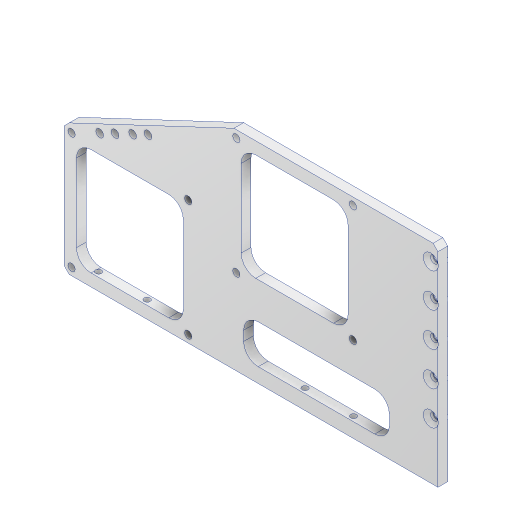
# Autodesk Inventor part: 사이드프레임
Saved by Autodesk Inventor 2023.2 (Build 272271000, 271)
## iProperties
Created: 2022-12-27
Part Number: 사이드프레임
Material: 알루미늄 6061
Document SubType Name: Modeling
Designer: BAEK
Density: 2.7 g/cm^3
Appearance: 알루미늄 - 평지
Mass: 77.0688 g
Surface Area: 191.691 cm^2
Volume: 28.544 cm^3
Author: BAEK
Autodesk Inventor part; units mm, degrees
ref_plane "YZ Plane" through (0, 0, 0) normal (1, 0, 0) x (0, 1, 0)
ref_plane "XZ Plane" through (0, 0, 0) normal (0, 1, 0) x (-1, 0, 0)
ref_plane "XY Plane" through (0, 0, 0) normal (0, 0, 1) x (1, 0, 0)
sketch "스케치1" plane through (0, 0, 0) normal (0, 0, 1) x (1, 0, 0)
  line L0 (27, 25) -> (25, 27)
  line L1 (-25, 27) -> (25, 27)
  line L2 (-25, 27) -> (-27, 25)
  line L3 (-27, -25) -> (-27, 25)
  line L4 (-27, -25) -> (-25, -27)
  line L5 (25, -27) -> (-25, -27)
  line L6 (25, -27) -> (27, -25)
  line L7 (27, 25) -> (27, -25)
  circle A0 centre (24, 24) radius 1.5
  circle A1 centre (-24, 24) radius 1.5
  circle A2 centre (24, -24) radius 1.5
  circle A3 centre (-24, -24) radius 1.5
  line L8 (-22, 22) -> (22, 22)
  line L9 (22, 22) -> (22, -22)
  line L10 (22, -22) -> (-22, -22)
  line L11 (-22, -22) -> (-22, 22)
  line L12 (-22, 22) -> (-17, 22)
  line L13 (-17, 22) -> (-17, 17)
  line L14 (-17, 17) -> (-22, 17)
  line L15 (-22, 17) -> (-22, 22)
  line L16 (22, 22) -> (17, 22)
  line L17 (17, 22) -> (17, 17)
  line L18 (17, 17) -> (22, 17)
  line L19 (22, 17) -> (22, 22)
  line L20 (-22, -22) -> (-17, -22)
  line L21 (-17, -22) -> (-17, -17)
  line L22 (-17, -17) -> (-22, -17)
  line L23 (-22, -17) -> (-22, -22)
  line L24 (22, -22) -> (17, -22)
  line L25 (17, -22) -> (17, -17)
  line L26 (17, -17) -> (22, -17)
  line L27 (22, -17) -> (22, -22)
  circle A4 centre (-17, 17) radius 5
  circle A5 centre (17, 17) radius 5
  circle A6 centre (17, -17) radius 5
  circle A7 centre (-17, -17) radius 5
  line L28 (0, -22) -> (0, 22)
  line L29 (22, 0) -> (-22, 0)
  point P0 (0, 0)
  point P1 (0, 0)
  dimension "d0" = 5
  dimension "d1" = 5
  dimension "d2" = 5
  dimension "d3" = 5
  dimension "d4" = 5
  dimension "d5" = 5
  dimension "d6" = 5
  dimension "d7" = 5
  constraints: 60 end point, 8 parallel, 5 midpoint, 4 centre point, 4 coincident, 4 horizontal, 4 horizontal alignment, 4 perpendicular, 8 other
  measures "d0" distance of L14.start L14.end
  measures "d1" distance of L13.start L14.start
  measures "d2" distance of L18.end L18.start
  measures "d3" distance of L18.start L16.end
  measures "d4" distance of L22.end L22.start
  measures "d5" distance of L22.start L21.start
  measures "d6" distance of L26.start L26.end
  measures "d7" distance of L24.end L26.start
extrude "돌출1" add sketch "스케치1" along normal blind 4
sketch "스케치3" plane through (0, 0, 4) normal (0, 0, 1) x (1, 0, 0)
  line L0 (27, -25) -> (27, 25) projected
  line L1 (27, 25) -> (25, 27) projected
  line L2 (25, 27) -> (-25, 27) projected
  line L3 (-25, 27) -> (-27, 25) projected
  line L4 (-27, 25) -> (-27, -25) projected
  line L5 (-27, -25) -> (-25, -27) projected
  line L6 (-25, -27) -> (25, -27) projected
  line L7 (25, -27) -> (27, -25) projected
  line L8 (22, 22) -> (22, -22) projected
  line L9 (22, -22) -> (-22, -22) projected
  line L10 (-22, -22) -> (-22, 22) projected
  line L11 (-22, 22) -> (22, 22) projected
  circle A0 centre (-24, -24) radius 1.5 projected
  circle A1 centre (24, -24) radius 1.5 projected
  circle A2 centre (24, 24) radius 1.5 projected
  circle A3 centre (-24, 24) radius 1.5 projected
  line L12 (45.8307, 54) -> (89.8307, 54)
  line L13 (42.8307, 59) -> (92.8307, 59)
  line L14 (45.8307, 54) -> (50.8307, 54)
  circle A4 centre (50.8307, 49) radius 5
  line L15 (50.8307, 49) -> (45.8307, 49)
  line L16 (45.8307, 49) -> (45.8307, 54)
  circle A5 centre (43.8307, 56) radius 1.5
  line L17 (42.8307, 59) -> (40.8307, 57)
  line L18 (45.8307, 10) -> (45.8307, 54)
  line L19 (40.8307, 7) -> (40.8307, 57)
  line L20 (50.8307, 54) -> (50.8307, 49)
  line L21 (40.8307, 7) -> (42.8307, 5)
  line L22 (92.8307, 5) -> (42.8307, 5)
  line L23 (92.8307, 5) -> (94.8307, 7)
  circle A6 centre (91.8307, 8) radius 1.5
  circle A7 centre (43.8307, 8) radius 1.5
  line L24 (89.8307, 10) -> (45.8307, 10)
  line L25 (84.8307, 15) -> (89.8307, 15)
  line L26 (89.8307, 10) -> (84.8307, 10)
  line L27 (89.8307, 15) -> (89.8307, 10)
  circle A8 centre (84.8307, 15) radius 5
  line L28 (50.8307, 10) -> (50.8307, 15)
  line L29 (50.8307, 15) -> (45.8307, 15)
  circle A9 centre (50.8307, 15) radius 5
  line L30 (45.8307, 10) -> (50.8307, 10)
  line L31 (45.8307, 15) -> (45.8307, 10)
  line L32 (84.8307, 10) -> (84.8307, 15)
  line L33 (94.8307, 57) -> (92.8307, 59)
  line L34 (89.8307, 54) -> (89.8307, 10)
  line L35 (94.8307, 57) -> (94.8307, 7)
  line L36 (84.8307, 54) -> (84.8307, 49)
  circle A10 centre (84.8307, 49) radius 5
  line L37 (84.8307, 49) -> (89.8307, 49)
  line L38 (89.8307, 54) -> (84.8307, 54)
  line L39 (89.8307, 49) -> (89.8307, 54)
  circle A11 centre (91.8307, 56) radius 1.5
  line L40 (45.8307, 32) -> (89.8307, 32)
  line L41 (67.8307, 54) -> (67.8307, 10)
  line L42 (0, 0) -> (67.8307, 32)
  line L43 (67.8307, 32) -> (67.8307, 0)
  line L44 (25, 27) -> (-25, 27) projected
  line L45 (-25, 27) -> (42.8307, 59)
  line L46 (-25, -27) -> (25, -27) projected
  line L47 (25, -27) -> (92.8307, 5)
  point P0 (67.8307, 32)
  point P1 (67.8307, 32)
  point P2 (89.8307, 49)
  point P3 (89.8307, 15)
  dimension "d41" = 5
  dimension "d42" = 5
  dimension "d43" = 5
  dimension "d44" = 5
  dimension "d45" = 5
  dimension "d46" = 5
  dimension "d47" = 5
  dimension "d48" = 5
  dimension "d49" = 5
  dimension "d50" = 24
  dimension "d51" = 48
  dimension "d52" = 48
  dimension "d53" = 48
  dimension "d54" = 75
  dimension "d55" = 32
  constraints: 68 end point, 9 parallel, 6 midpoint, 5 coincident, 5 horizontal alignment, 4 centre point, 4 horizontal, 4 perpendicular, 1 vertical, 8 other
  measures "d41" distance of L15.start L15.end
  measures "d42" distance of L20.start L15.start
  measures "d43" distance of L37.end L36.end
  measures "d44" distance of L36.end L36.start
  measures "d45" distance of L31.start L28.end
  measures "d46" distance of L28.end L28.start
  measures "d47" distance of L25.start L27.start
  measures "d48" distance of L26.end L25.start
  measures "d49" distance between parallel lines of L19 L18
  measures "d50" horizontal distance of point (67.831, 32) A5.centre
  measures "d51" distance of A11.centre A5.centre
  measures "d52" distance of A5.centre A7.centre
  measures "d53" distance of A6.centre A7.centre
  measures "d54" distance of L42.start L42.end
  measures "d55" distance of L42.end L43.end
extrude "돌출4" add sketch "스케치3" against normal blind 4 contours L0 L42 L19 L21 L22 L47 L7 | L0 L1 L2 L45 L17 L19 L42 | L42 L18 L24 L43 L22 L21 L19 | L19 L17 L13 L33 L35 L23 L22 L43 L24 L27 L34 L12 L16 L18 L42
sketch "스케치6" plane through (0, 0, 4) normal (0, 0, 1) x (1, 0, 0)
  circle A0 centre (43.8307, 8) radius 1.5 projected
  circle A1 centre (43.8307, 56) radius 1.5 projected
  circle A2 centre (91.8307, 8) radius 1.5 projected
  circle A3 centre (91.8307, 56) radius 1.5 projected
  line L0 (89.8307, 10) -> (45.8307, 10) projected
  line L1 (45.8307, 10) -> (45.8307, 54) projected
  line L2 (45.8307, 54) -> (89.8307, 54) projected
  line L3 (89.8307, 54) -> (89.8307, 10) projected
  line L4 (25, -27) -> (92.8307, 5) projected
  line L5 (92.8307, 5) -> (94.8307, 7) projected
  line L6 (94.8307, 7) -> (94.8307, 57) projected
  line L7 (94.8307, 57) -> (92.8307, 59) projected
  line L8 (92.8307, 59) -> (42.8307, 59) projected
  line L9 (42.8307, 59) -> (-25, 27) projected
  line L10 (-25, 27) -> (-27, 25) projected
  line L11 (-27, 25) -> (-27, -25) projected
  line L12 (-27, -25) -> (-25, -27) projected
  line L13 (-25, -27) -> (25, -27) projected
  line L14 (22, 22) -> (22, -22) projected
  line L15 (22, -22) -> (-22, -22) projected
  line L16 (-22, -22) -> (-22, 22) projected
  line L17 (-22, 22) -> (22, 22) projected
  circle A4 centre (-24, -24) radius 1.5 projected
  circle A5 centre (24, -24) radius 1.5 projected
  circle A6 centre (24, 24) radius 1.5 projected
  circle A7 centre (-24, 24) radius 1.5 projected
  line L18 (-25, -27) -> (25, -27) projected
  line L19 (25, -27) -> (94.8307, -27)
  line L20 (94.8307, -27) -> (94.8307, 7)
  point P0 (0, 0)
  constraints: 4 end point, 1 horizontal, 1 perpendicular
extrude "돌출5" add sketch "스케치6" against normal blind 4 contours L4 L5 L20 L19
sketch "스케치9" plane through (0, 0, 4) normal (0, 0, 1) x (1, 0, 0)
  circle A0 centre (43.8307, 8) radius 1.5 projected
  circle A1 centre (43.8307, 56) radius 1.5 projected
  circle A2 centre (91.8307, 8) radius 1.5 projected
  circle A3 centre (91.8307, 56) radius 1.5 projected
  line L0 (89.8307, 10) -> (45.8307, 10) projected
  line L1 (45.8307, 10) -> (45.8307, 54) projected
  line L2 (45.8307, 54) -> (89.8307, 54) projected
  line L3 (89.8307, 54) -> (89.8307, 10) projected
  line L4 (94.8307, -27) -> (94.8307, 57) projected
  line L5 (94.8307, 57) -> (92.8307, 59) projected
  line L6 (92.8307, 59) -> (42.8307, 59) projected
  line L7 (42.8307, 59) -> (-25, 27) projected
  line L8 (-25, 27) -> (-27, 25) projected
  line L9 (-27, 25) -> (-27, -25) projected
  line L10 (-27, -25) -> (-25, -27) projected
  line L11 (-25, -27) -> (94.8307, -27) projected
  line L12 (22, 22) -> (22, -22) projected
  line L13 (22, -22) -> (-22, -22) projected
  line L14 (-22, -22) -> (-22, 22) projected
  line L15 (-22, 22) -> (22, 22) projected
  circle A4 centre (-24, -24) radius 1.5 projected
  circle A5 centre (24, -24) radius 1.5 projected
  circle A6 centre (24, 24) radius 1.5 projected
  circle A7 centre (-24, 24) radius 1.5 projected
  line L16 (94.8307, 57) -> (94.8307, -27) projected
  line L17 (94.8307, -27) -> (126.8307, -27)
  line L18 (126.8307, -27) -> (126.8307, 59)
  line L19 (126.8307, 59) -> (94.8307, 59)
  line L20 (94.8307, 59) -> (94.8307, -27)
  line L21 (94.8307, 59) -> (92.8307, 59)
  point P0 (0, 0)
  dimension "d60" = 32
  constraints: 10 end point, 2 parallel, 1 collinear, 1 horizontal, 1 perpendicular
  measures "d60" distance of L19.end L18.end
extrude "돌출6" add sketch "스케치9" against normal blind 4 contours L4 L20 L19 L18 L17 | L5 L21 L20
sketch "스케치10" plane through (0, 0, 4) normal (0, 0, 1) x (1, 0, 0)
  line L0 (-25, 27) -> (42.8307, 59) projected
  line L1 (-25, 27) -> (-20.0258, 29.3467)
  line L2 (-20.0258, 29.3467) -> (-17.4658, 23.9202)
  line L3 (-17.4658, 23.9202) -> (15.093, 39.2802)
  line L4 (15.093, 39.2802) -> (12.533, 44.7067)
  line L5 (-18.7458, 26.6334) -> (13.813, 41.9934) construction
  circle A0 centre (-12.4149, 29.6201) radius 1.6
  circle A1 centre (-6.084, 32.6068) radius 1.6
  circle A2 centre (1.1512, 36.0201) radius 1.6
  circle A3 centre (7.4821, 39.0068) radius 1.6
  point P0 (0, 0)
  dimension "d63" = 5.5
  dimension "d64" = 6
  dimension "d65" = 90
  dimension "d66" = 36
  dimension "d68" = 3.2
  dimension "d69" = 3.2
  dimension "d70" = 3.2
  dimension "d71" = 3.2
  dimension "d72" = 7
  dimension "d73" = 7
  dimension "d74" = 7
  dimension "d75" = 7
  constraints: 10 end point, 6 point on line, 4 centre point, 2 midpoint, 1 perpendicular
  measures "d63" distance of L0.start L1.end
  measures "d64" distance of L1.end L2.end
  measures "d65" angle of L0 L2
  measures "d66" distance of L2.end L3.end
  measures "d68" diameter of A0
  measures "d69" diameter of A1
  measures "d70" diameter of A2
  measures "d71" diameter of A3
  measures "d72" distance from line of L2 A0.centre
  measures "d73" distance from line of L4 A3.centre
  measures "d74" distance of A3.centre A2.centre
  measures "d75" distance of A0.centre A1.centre
extrude "돌출7" cut sketch "스케치10" against normal blind 4 contours A0 | A1 | A2 | A3
fillet "모깎기1" radius 6 8 edges at (45.8307, 10, 2) (45.8307, 54, 2) (89.8307, 54, 2) (89.8307, 10, 2) (22, 22, 2) (22, -22, 2) (-22, -22, 2) (-22, 22, 2)
sketch "스케치11" plane through (0, 0, 4) normal (0, 0, 1) x (1, 0, 0)
  circle A0 centre (1.1512, 36.0201) radius 1.6 projected
  circle A1 centre (-6.084, 32.6068) radius 1.6 projected
  circle A2 centre (7.4821, 39.0068) radius 1.6 projected
  circle A3 centre (-12.4149, 29.6201) radius 1.6 projected
  circle A4 centre (43.8307, 8) radius 1.5 projected
  circle A5 centre (43.8307, 56) radius 1.5 projected
  circle A6 centre (91.8307, 8) radius 1.5 projected
  circle A7 centre (91.8307, 56) radius 1.5 projected
  line L0 (83.8307, 10) -> (51.8307, 10) projected
  arc A8 (45.8307, 16) -> (51.8307, 10) centre (51.8307, 16) ccw projected
  line L1 (45.8307, 16) -> (45.8307, 48) projected
  arc A9 (51.8307, 54) -> (45.8307, 48) centre (51.8307, 48) ccw projected
  line L2 (51.8307, 54) -> (83.8307, 54) projected
  arc A10 (89.8307, 48) -> (83.8307, 54) centre (83.8307, 48) ccw projected
  line L3 (89.8307, 48) -> (89.8307, 16) projected
  arc A11 (83.8307, 10) -> (89.8307, 16) centre (83.8307, 16) ccw projected
  line L4 (126.8307, 59) -> (42.8307, 59) projected
  line L5 (42.8307, 59) -> (-25, 27) projected
  line L6 (-25, 27) -> (-27, 25) projected
  line L7 (-27, 25) -> (-27, -25) projected
  line L8 (-27, -25) -> (-25, -27) projected
  line L9 (-25, -27) -> (126.8307, -27) projected
  line L10 (126.8307, -27) -> (126.8307, 59) projected
  line L11 (22, 16) -> (22, -16) projected
  arc A12 (16, -22) -> (22, -16) centre (16, -16) ccw projected
  line L12 (16, -22) -> (-16, -22) projected
  arc A13 (-22, -16) -> (-16, -22) centre (-16, -16) ccw projected
  line L13 (-22, -16) -> (-22, 16) projected
  arc A14 (-16, 22) -> (-22, 16) centre (-16, 16) ccw projected
  line L14 (-16, 22) -> (16, 22) projected
  arc A15 (22, 16) -> (16, 22) centre (16, 16) ccw projected
  circle A16 centre (-24, -24) radius 1.5 projected
  circle A17 centre (24, -24) radius 1.5 projected
  circle A18 centre (24, 24) radius 1.5 projected
  circle A19 centre (-24, 24) radius 1.5 projected
  line L15 (126.8307, 59) -> (120.8307, 59)
  line L16 (120.8307, 59) -> (120.8307, -11)
  line L17 (120.8307, -11) -> (126.8307, -11)
  line L18 (126.8307, -11) -> (126.8307, 59)
  line L19 (126.8307, 59) -> (42.8307, 59) projected
  line L20 (123.8307, 59) -> (123.8307, -11) construction
  circle A20 centre (123.8307, 52) radius 1.6
  circle A21 centre (123.8307, 38) radius 1.6
  circle A22 centre (123.8307, 24) radius 1.6
  circle A23 centre (123.8307, 10) radius 1.6
  circle A24 centre (123.8307, -4) radius 1.6
  point P0 (0, 0)
  dimension "d79" = 6
  dimension "d80" = 70
  dimension "d81" = 3.2
  dimension "d82" = 3.2
  dimension "d83" = 3.2
  dimension "d84" = 3.2
  dimension "d85" = 3.2
  dimension "d86" = 7
  dimension "d87" = 14
  dimension "d88" = 7
  dimension "d89" = 14
  dimension "d90" = 14
  constraints: 10 end point, 5 centre point, 5 point on line, 2 midpoint, 2 parallel, 1 horizontal, 1 perpendicular
  measures "d79" distance of L17.end L16.end
  measures "d80" distance of L15.end L16.end
  measures "d81" diameter of A20
  measures "d82" diameter of A21
  measures "d83" diameter of A22
  measures "d84" diameter of A23
  measures "d85" diameter of A24
  measures "d86" distance from line of L4 A20.centre
  measures "d87" distance of A20.centre A21.centre
  measures "d88" distance of L20.end A24.centre
  measures "d89" distance of A24.centre A23.centre
  measures "d90" distance of A22.centre A23.centre
extrude "돌출8" cut sketch "스케치11" against normal blind 4 contours A20 | A21 | A22 | A23 | A24
sketch "스케치12" plane through (0, 0, 4) normal (0, 0, 1) x (1, 0, 0)
  circle A0 centre (123.8307, 24) radius 1.6 projected
  circle A1 centre (123.8307, 10) radius 1.6 projected
  circle A2 centre (123.8307, 38) radius 1.6 projected
  circle A3 centre (123.8307, -4) radius 1.6 projected
  circle A4 centre (123.8307, 52) radius 1.6 projected
  circle A5 centre (1.1512, 36.0201) radius 1.6 projected
  circle A6 centre (-6.084, 32.6068) radius 1.6 projected
  circle A7 centre (7.4821, 39.0068) radius 1.6 projected
  circle A8 centre (-12.4149, 29.6201) radius 1.6 projected
  circle A9 centre (43.8307, 8) radius 1.5 projected
  circle A10 centre (43.8307, 56) radius 1.5 projected
  circle A11 centre (91.8307, 8) radius 1.5 projected
  circle A12 centre (91.8307, 56) radius 1.5 projected
  line L0 (83.8307, 10) -> (51.8307, 10) projected
  arc A13 (45.8307, 16) -> (51.8307, 10) centre (51.8307, 16) ccw projected
  line L1 (45.8307, 16) -> (45.8307, 48) projected
  arc A14 (51.8307, 54) -> (45.8307, 48) centre (51.8307, 48) ccw projected
  line L2 (51.8307, 54) -> (83.8307, 54) projected
  arc A15 (89.8307, 48) -> (83.8307, 54) centre (83.8307, 48) ccw projected
  line L3 (89.8307, 48) -> (89.8307, 16) projected
  arc A16 (83.8307, 10) -> (89.8307, 16) centre (83.8307, 16) ccw projected
  line L4 (126.8307, 59) -> (42.8307, 59) projected
  line L5 (42.8307, 59) -> (-25, 27) projected
  line L6 (-25, 27) -> (-27, 25) projected
  line L7 (-27, 25) -> (-27, -25) projected
  line L8 (-27, -25) -> (-25, -27) projected
  line L9 (-25, -27) -> (126.8307, -27) projected
  line L10 (126.8307, -27) -> (126.8307, 59) projected
  line L11 (22, 16) -> (22, -16) projected
  arc A17 (16, -22) -> (22, -16) centre (16, -16) ccw projected
  line L12 (16, -22) -> (-16, -22) projected
  arc A18 (-22, -16) -> (-16, -22) centre (-16, -16) ccw projected
  line L13 (-22, -16) -> (-22, 16) projected
  arc A19 (-16, 22) -> (-22, 16) centre (-16, 16) ccw projected
  line L14 (-16, 22) -> (16, 22) projected
  arc A20 (22, 16) -> (16, 22) centre (16, 16) ccw projected
  circle A21 centre (-24, -24) radius 1.5 projected
  circle A22 centre (24, -24) radius 1.5 projected
  circle A23 centre (24, 24) radius 1.5 projected
  circle A24 centre (-24, 24) radius 1.5 projected
  line L15 (126.8307, 59) -> (126.8307, -27) projected
  line L16 (126.8307, -27) -> (76.8307, -27)
  line L17 (99.3307, -7) -> (126.8307, -7)
  line L18 (126.8307, -7) -> (126.8307, -27)
  line L19 (76.8307, -7) -> (76.8307, -13)
  line L20 (46.8307, -5) -> (106.8307, -5)
  line L21 (106.8307, -5) -> (106.8307, -21)
  line L22 (106.8307, -21) -> (46.8307, -21)
  line L23 (46.8307, -21) -> (46.8307, -5)
  line L24 (46.8307, -5) -> (106.8307, -21) construction
  line L25 (106.8307, -5) -> (46.8307, -21) construction
  line L26 (76.8307, -27) -> (76.8307, -21)
  line L27 (76.8307, -13) -> (76.8307, -7)
  point P0 (0, 0)
  dimension "d93" = 50
  dimension "d94" = 20
  dimension "d95" = 6
  dimension "d96" = 60
  dimension "d97" = 16
  constraints: 24 end point, 5 parallel, 4 midpoint, 3 perpendicular, 2 horizontal, 1 point on line
  measures "d93" distance of L19.start L17.end
  measures "d94" distance of L16.end L19.start
  measures "d95" distance of L19.start L19.end
  measures "d96" distance of L21.end L22.end
  measures "d97" distance of L20.end L21.end
extrude "돌출9" cut sketch "스케치12" against normal blind 4 contours L21 L22 L23 L20
fillet "모깎기2" radius 6 4 edges at (46.8307, -5, 2) (46.8307, -21, 2) (106.8307, -21, 2) (106.8307, -5, 2)
sketch "스케치13" plane through (-25, -27, 0) normal (0, -1, 0) x (1, 0, 0)
  line L0 (-2, 0) -> (-2, 4) projected
  line L1 (-2, 2) -> (151.8307, 2) construction
  circle A0 centre (10.111, 2) radius 1.25
  circle A1 centre (30.111, 2) radius 1.25
  circle A2 centre (60.111, 2) radius 1.25
  circle A3 centre (75.111, 2) radius 1.25
  circle A4 centre (95.111, 2) radius 1.25
  circle A5 centre (115.111, 2) radius 1.25
  circle A6 centre (140.111, 2) radius 1.25
  point P0 (25, 0)
  dimension "d101" = 2.5
  dimension "d103" = 2.5
  dimension "d104" = 12.111
  dimension "d105" = 20
  dimension "d108" = 20
  dimension "d109" = 20
  dimension "d110" = 25
  dimension "d111" = 30
  dimension "d112" = 15
  constraints: 7 centre point, 5 equal radius, 1 midpoint, 10 other
  measures "d101" diameter of A0
  measures "d103" diameter of A1
  measures "d104" distance of point (-2, 2) A0.centre
  measures "d105" distance of A0.centre A1.centre
  measures "d108" distance of A4.centre A5.centre
  measures "d109" distance of A3.centre A4.centre
  measures "d110" distance of A5.centre A6.centre
  measures "d111" distance of A1.centre A2.centre
  measures "d112" distance of A2.centre A3.centre
extrude "돌출10" cut sketch "스케치13" against normal blind 6
chamfer "모따기1" distance 2 angle 45 1 edges at (126.8307, 59, 2)
chamfer "모따기2" distance 1.5 angle 45 5 edges at (122.2307, 52, 0) (122.2307, 38, 0) (122.2307, 24, 0) (122.2307, 10, 0) (122.2307, -4, 0)
chamfer "모따기3" distance 1.5 angle 45 5 edges at (122.2307, 52, 4) (122.2307, 38, 4) (122.2307, 24, 4) (122.2307, 10, 4) (122.2307, -4, 4)
sketch "스케치14" plane through (42.8307, 59, 4) normal (0, 1, 0) x (1, 0, 0)
  line L0 (82, 4) -> (82, 0) projected
  line L1 (0, 4) -> (82, 4) projected
  line L2 (0, 0) -> (0, 4) projected
  line L3 (82, 0) -> (0, 0) projected
  circle A0 centre (67.448, 2) radius 1.25
  line L4 (84, 0) -> (84, 4) projected
  circle A1 centre (46.398, 2) radius 1.25
  circle A2 centre (25.348, 2) radius 1.25
  point P0 (-42.8307, 4)
  point P1 (84, 2)
  dimension "d118" = 2.5
  dimension "d119" = 16.552
  dimension "d120" = 2.5
  dimension "d121" = 2.5
  dimension "d122" = 21.05
  dimension "d123" = 21.05
  constraints: 3 centre point, 1 midpoint
  measures "d118" diameter of A0
  measures "d119" distance of point (84, 2) A0.centre
  measures "d120" diameter of A1
  measures "d121" diameter of A2
  measures "d122" distance of A0.centre A1.centre
  measures "d123" distance of A1.centre A2.centre
